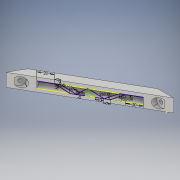
# Autodesk Inventor part: 120deg_Tslot_Gusset
Saved by Autodesk Inventor 2019.4 (Build 234330000, 330)
## iProperties
Created: 2020-02-22
Part Number: 120deg_Tslot_Gusset
Material: Generic
Document SubType Name: Modeling
Designer: Jorian Brusind
Density: 1 g/cm^3
Appearance: Default
Author: Jorian Brusind
Autodesk Inventor part; units mm, degrees
ref_plane "YZ Plane" through (0, 0, 0) normal (1, 0, 0) x (0, 1, 0)
ref_plane "XZ Plane" through (0, 0, 0) normal (0, 1, 0) x (-1, 0, 0)
sketch "Sketch1" plane through (0, 0, 0) normal (0, 1, 0) x (-1, 0, 0)
  line L0 (0.3427, -0.4489) -> (100.3427, -0.4489)
  line L1 (0.3427, -0.4489) -> (100.3427, -0.4489) construction
  line L2 (100.3427, -0.4489) -> (150.3427, 86.1536)
  line L3 (0.3427, -0.4489) -> (0.3427, 9.5511)
  line L4 (150.3427, 86.1536) -> (141.6824, 91.1536)
  line L5 (150.3427, 86.1536) -> (160.3427, 86.1536) construction
  line L6 (0.3427, 9.5511) -> (10.3427, 9.5511)
  line L7 (0.3427, 9.5511) -> (-14.6573, 9.5511)
  line L8 (141.6824, 91.1536) -> (136.3686, 82.6823)
  line L9 (141.6824, 91.1536) -> (148.759, 104.3794)
  line L10 (136.3686, 82.6823) -> (10.3427, 9.5511)
  line L11 (148.759, 104.3794) -> (-14.6573, 9.5511)
  dimension "d2" = 100
  dimension "d3" = 0
  dimension "d4" = 100
  dimension "d5" = 120
  dimension "d6" = 10
  dimension "d7" = 10
  dimension "d8" = 150
  dimension "d9" = 10
  dimension "d10" = 15
  dimension "d11" = 10
  dimension "d12" = 15
  constraints: 24 end point, 5 horizontal, 2 equal length, 1 parallel, 1 vertical
  measures "d2" distance of L0.start L0.end
  measures "d3" distance between parallel lines of L0 L1
  measures "d4" distance of L0.end L2.end
  measures "d5" angle of L2 L0
  measures "d6" distance of L0.start L3.end
  measures "d7" distance of L2.end L4.end
  measures "d8" angle of L5 L4
  measures "d9" distance of L3.end L6.end
  measures "d10" distance of L3.end L7.end
  measures "d11" distance of L4.end L8.end
  measures "d12" distance of L4.end L9.end
extrude "Extrusion1" add sketch "Sketch1" along normal blind 20 contours L7 L11 L9 L8 L10 L6
ref_plane "Work Plane1" through (0, 0, 15) normal (0, 0, 1) x (1, 0, 0)
ref_plane "Work Plane3" through (-144.3504, 0, 106.7383) normal (-0.8817208, 0, -0.4717715) x (-0.4717715, 0, 0.8817208)
sketch "Sketch7" plane through (-144.3504, 0, 106.7383) normal (-0.8817208, 0, -0.4717715) x (-0.4717715, 0, 0.8817208)
  line L0 (0, 0) -> (0, 20) projected
  line L1 (0, 0) -> (0, 5)
  line L2 (0, 5) -> (-5, 5)
  line L3 (-24.9763, 0) -> (-24.9763, 20) projected
  line L4 (-24.9763, 20) -> (-24.9763, 15)
  line L5 (-24.9763, 15) -> (-19.9763, 15)
  line L6 (-19.9763, 15) -> (-5, 15)
  line L7 (-5, 15) -> (-5, 5)
  line L8 (-5, 5) -> (-19.9763, 5)
  line L9 (-19.9763, 5) -> (-19.9763, 15)
  point P0 (-162.2138, 0)
  dimension "d38" = 5
  dimension "d39" = 5
  dimension "d40" = 5
  dimension "d41" = 5
  constraints: 16 end point, 3 perpendicular, 2 parallel, 2 point on line, 1 horizontal
  measures "d38" distance of L0.start L1.end
  measures "d39" distance of L1.end L2.end
  measures "d40" distance of L3.end L4.end
  measures "d41" distance of L4.end L5.end
extrude "Extrusion6" cut sketch "Sketch7" against normal blind 10
ref_plane "Work Plane4" through (14.6573, 0, 14.5511) normal (0, 0, -1) x (-1, 0, 0)
sketch "Sketch8" plane through (14.6573, 0, 14.5511) normal (0, 0, -1) x (-1, 0, 0)
  line L0 (0, 0) -> (0, 20) projected
  line L1 (0, 20) -> (0, 15)
  line L2 (0, 15) -> (5, 15)
  line L3 (25, 0) -> (25, 20) projected
  line L4 (25, 0) -> (25, 5)
  line L5 (25, 0) -> (30, 0) construction
  line L6 (25, 5) -> (20, 5)
  line L7 (5, 15) -> (20, 15)
  line L8 (20, 15) -> (20, 5)
  line L9 (20, 5) -> (5, 5)
  line L10 (5, 5) -> (5, 15)
  point P0 (14.6573, 0)
  dimension "d45" = 5
  dimension "d46" = 5
  dimension "d47" = 5
  dimension "d48" = 90
  dimension "d49" = 5
  constraints: 18 end point, 4 perpendicular, 2 horizontal, 2 parallel, 1 collinear, 1 point on line
  measures "d45" distance of L0.end L1.end
  measures "d46" distance of L1.end L2.end
  measures "d47" distance of L3.start L4.end
  measures "d48" angle of L5 L4
  measures "d49" distance of L4.end L6.end
extrude "Extrusion7" cut sketch "Sketch8" against normal blind 10
sketch "Sketch9" plane through (-144.3504, 0, 106.7383) normal (0.8817208, 0, 0.4717715) x (0.4717715, 0, -0.8817208)
  line L0 (8.0879, 5) -> (8.0879, 15) projected
  line L1 (8.0879, 10) -> (14.0321, 10)
  line L2 (19.9763, 5) -> (8.0879, 5) projected
  circle A0 centre (14.0321, 10) radius 7.5
  point P0 (162.2138, 0)
  dimension "d52" = 15
  constraints: 2 end point, 1 centre point, 1 coincident, 1 midpoint, 1 parallel
  measures "d52" diameter of A0
extrude "Extrusion8" cut sketch "Sketch9" along normal blind 10 contours A0 L0 | L0 A0 L2 | L2 A0 picked at (12.0507, 6.6667)
sketch "Sketch10" plane through (-144.3504, 0, 106.7383) normal (0.8817208, 0, 0.4717715) x (0.4717715, 0, -0.8817208)
  arc A0 (19.6223, 15) -> (8.4419, 15) centre (14.0321, 10) ccw projected
  circle A1 centre (14.0321, 10) radius 2.75
  point P0 (162.2138, 0)
  dimension "d55" = 5.5
  constraints: 1 centre point, 1 coincident
  measures "d55" diameter of A1
extrude "Extrusion9" cut sketch "Sketch10" against normal blind 5
sketch "Sketch11" plane through (14.6573, 0, 14.5511) normal (0, 0, 1) x (1, 0, 0)
  line L0 (-20, 15) -> (-8.6164, 15) projected
  line L1 (-14.3082, 15) -> (-14.3082, 10)
  line L2 (-14.3082, 15) -> (-9.3082, 15) construction
  circle A0 centre (-14.3082, 10) radius 7.5
  point P0 (-14.6573, 0)
  dimension "d58" = 90
  dimension "d59" = 15
  constraints: 4 end point, 1 centre point, 1 coincident, 1 horizontal, 1 midpoint, 1 perpendicular
  measures "d58" angle of L1 L2
  measures "d59" diameter of A0
extrude "Extrusion10" cut sketch "Sketch11" along normal blind 10
sketch "Sketch12" plane through (14.6573, 0, 14.5511) normal (0, 0, 1) x (1, 0, 0)
  arc A0 (-8.718, 15) -> (-19.8984, 15) centre (-14.3082, 10) ccw projected
  circle A1 centre (-14.3082, 10) radius 2.75
  point P0 (-14.6573, 0)
  dimension "d62" = 5.5
  constraints: 1 centre point, 1 coincident
  measures "d62" diameter of A1
extrude "Extrusion11" cut sketch "Sketch12" against normal blind 5
sketch "Sketch13" plane through (14.6573, 0, 9.5511) normal (0.5019038, 0, 0.8649235) x (0.8649235, 0, -0.5019038)
  line L0 (-188.9373, 20) -> (0, 20) projected
  line L1 (-94.4687, 20) -> (-154.4687, 20)
  line L2 (-154.4687, 20) -> (-154.4687, 15)
  line L3 (-188.9373, 0) -> (0, 0) projected
  line L4 (-94.4687, 0) -> (-34.4687, 0)
  line L5 (-34.4687, 0) -> (-34.4687, 5)
  line L6 (-34.4687, 5) -> (-154.4687, 5)
  line L7 (-154.4687, 5) -> (-154.4687, 15)
  line L8 (-154.4687, 15) -> (-34.4687, 15)
  line L9 (-34.4687, 15) -> (-34.4687, 5)
  point P0 (-7.8837, 0)
  dimension "d65" = 60
  dimension "d66" = 5
  dimension "d67" = 60
  dimension "d68" = 5
  constraints: 16 end point, 2 midpoint, 2 parallel, 2 perpendicular, 2 point on line, 1 horizontal, 1 vertical
  measures "d65" distance of L1.start L1.end
  measures "d66" distance of L1.end L2.end
  measures "d67" distance of L4.start L4.end
  measures "d68" distance of L4.end L5.end
extrude "Extrusion12" cut sketch "Sketch13" against normal blind 15
sketch "Sketch14" plane through (14.6573, 0, 9.5511) normal (0.5019038, 0, 0.8649235) x (0.8649235, 0, -0.5019038)
  line L0 (-34.4687, 15) -> (-154.4687, 15) projected
  line L1 (-154.4687, 15) -> (-134.4687, 15)
  line L2 (-34.4687, 15) -> (-54.4687, 15)
  line L3 (-134.4687, 15) -> (-117.1482, 5)
  line L4 (-154.4687, 5) -> (-34.4687, 5) projected
  line L5 (-134.4687, 15) -> (-114.4687, 15) construction
  line L6 (-54.4687, 15) -> (-71.7892, 5)
  line L7 (-54.4687, 15) -> (-34.4687, 15) construction
  line L8 (-71.7892, 5) -> (-78.7892, 5)
  line L9 (-54.4687, 15) -> (-61.4687, 15)
  line L10 (-134.4687, 15) -> (-127.4687, 15)
  line L11 (-117.1482, 5) -> (-110.1482, 5)
  line L12 (-110.1482, 5) -> (-127.4687, 15)
  line L13 (-78.7892, 5) -> (-61.4687, 15)
  line L14 (-110.1482, 5) -> (-98.2306, 15)
  line L15 (-110.1482, 5) -> (-94.5909, 5) construction
  line L16 (-78.7892, 5) -> (-96.1097, 15)
  line L17 (-78.7892, 5) -> (-58.7892, 5) construction
  line L18 (-98.2306, 15) -> (-96.1097, 15)
  line L19 (-110.1482, 5) -> (-100.1482, 5)
  line L20 (-100.1482, 5) -> (-96.7451, 13.4266)
  line L21 (-78.7892, 5) -> (-88.7892, 5)
  line L22 (-88.7892, 5) -> (-96.7451, 13.4266)
  line L23 (-134.4687, 15) -> (-127.4687, 15)
  point P0 (-7.8837, 0)
  dimension "d71" = 20
  dimension "d72" = 20
  dimension "d73" = 30
  dimension "d74" = 150
  dimension "d75" = 7
  dimension "d76" = 7
  dimension "d77" = 7
  dimension "d78" = 7
  dimension "d79" = 40
  dimension "d80" = 150
  dimension "d81" = 10
  dimension "d82" = 10
  constraints: 44 end point, 12 point on line, 4 equal length, 4 horizontal, 2 collinear
  measures "d71" distance of L0.end L1.end
  measures "d72" distance of L0.start L2.end
  measures "d73" angle of L3 L5
  measures "d74" angle of L6 L7
  measures "d75" distance of L6.end L8.end
  measures "d76" distance of L2.end L9.end
  measures "d77" distance of L1.end L10.end
  measures "d78" distance of L3.end L11.end
  measures "d79" angle of L15 L14
  measures "d80" angle of L17 L16
  measures "d81" distance of L11.end L19.end
  measures "d82" distance of L8.end L21.end
body "Solid1"
